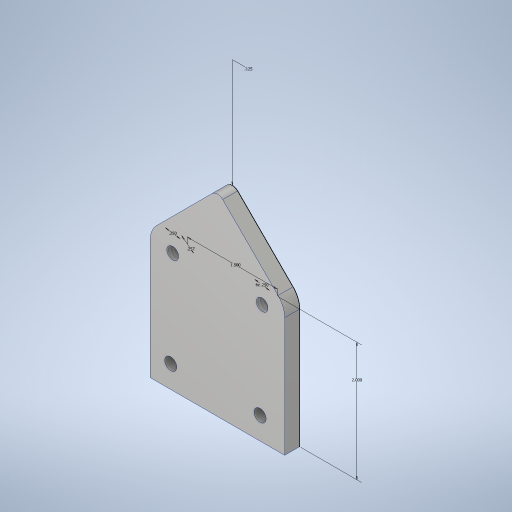
# Autodesk Inventor part: CL7-005a
Saved by Autodesk Inventor 2023.4 (Build 274418000, 418)
## iProperties
Created: 2025-03-17
Part Number: CL7-005a
Material: Aluminum 6061
Document SubType Name: Modeling
Designer: dlangdon
Density: 2.7 g/cm^3
Appearance: Aluminum - Flat
Author: dlangdon
Autodesk Inventor part; units mm, degrees
ref_plane "YZ Plane" through (0, 0, 0) normal (1, 0, 0) x (0, 1, 0)
ref_plane "XZ Plane" through (0, 0, 0) normal (0, 1, 0) x (-1, 0, 0)
ref_plane "XY Plane" through (0, 0, 0) normal (0, 0, 1) x (1, 0, 0)
sketch "Sketch1" plane through (0, 0, 0) normal (0, 0, 1) x (1, 0, 0)
  line L0 (-19.05, 0) -> (19.05, 0) construction
  circle A0 centre (-19.05, 0) radius 3.2639
  circle A1 centre (19.05, 0) radius 3.2639
  arc A2 (-25.8481, 6.7981) -> (-28.6639, 0) centre (-19.05, 0) ccw
  arc A3 (28.6639, 0) -> (25.8481, 6.7981) centre (19.05, 0) ccw
  line L1 (-28.6639, 0) -> (-28.6639, -50.8)
  line L2 (-28.6639, -50.8) -> (28.6639, -50.8)
  line L3 (28.6639, -50.8) -> (28.6639, 0)
  line L4 (-25.8481, 6.7981) -> (-2.2451, 30.401)
  line L5 (2.2451, 30.401) -> (25.8481, 6.7981)
  arc A4 (2.2451, 30.401) -> (-2.2451, 30.401) centre (0, 28.156) ccw
  point P0 (0, 0)
  point P1 (0, 0)
  dimension "d0" = 6.5278
  dimension "d1" = 38.1
  dimension "d2" = 6.35
  dimension "d3" = 6.35
  dimension "d4" = 50.8
  dimension "d5" = 3.175
  constraints: 12 end point, 6 point on circle, 6 tangent, 5 centre point, 5 coincident, 3 perpendicular, 2 vertical, 1 equal radius, 1 horizontal, 1 midpoint
  measures "d0" diameter of A0
  measures "d1" distance of L0.start L0.end
  measures "d2" radial gap between concentric circles of A0 A2
  measures "d3" radial gap between concentric circles of A1 A3
  measures "d4" distance from line of A1.centre L2
  measures "d5" radius of A4
extrude "Extrusion1" add sketch "Sketch1" along normal blind 6.35 contours A0 | A1 | L4 A4 L5 A3 L3 L2 L1 A2
sketch "Sketch2" plane through (0, 0, 6.35) normal (0, 0, 1) x (1, 0, 0)
  line L0 (-19.9009, -41.275) -> (18.1991, -41.275) construction
  line L1 (-28.6639, -50.8) -> (28.6639, -50.8) projected
  point P0 (0, 0)
  dimension "d8" = 38.1
  dimension "d9" = 9.525
  constraints: 2 coincident, 2 end point, 1 horizontal
  measures "d8" distance of L0.start L0.end
  measures "d9" distance between parallel lines of L0 L1
hole "Hole1" at (-19.9009, -41.275, 6.35) at (18.1991, -41.275, 6.35) direction (0, 0, -1) diameter 5.1054 end through all clearance for "Flat Head Machine Screw (82)" size "#10" standard "Ansi Unified Screw Threads"
hole "Hole2" at (-19.05, 0, 0) at (19.05, 0, 0) direction (0, 0, 1) diameter 4.9784 end through all thread size "1/4-20 UNC" class "2B" standard "ANSI Unified Screw Threads"
equation "\"d3\" = d2"
body "Solid1"
